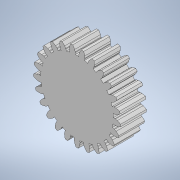
# Autodesk Inventor part: ｍ2歯数25ギア8t
Saved by Autodesk Inventor 2020.2 (Build 242310000, 310)
## iProperties
Created: 2020-02-29
Part Number: ｍ2歯数25ギア8t
Material: 一般
Document SubType Name: Modeling
Designer: aoyam
Density: 1 g/cm^3
Appearance: 既定
Author: aoyam
Autodesk Inventor part; units mm, degrees
ref_plane "YZ Plane" through (0, 0, 0) normal (1, 0, 0) x (0, 1, 0)
ref_plane "XZ Plane" through (0, 0, 0) normal (0, 1, 0) x (-1, 0, 0)
ref_plane "XY Plane" through (0, 0, 0) normal (0, 0, 1) x (1, 0, 0)
sketch "スケッチ1" plane through (0, 0, 0) normal (0, 0, 1) x (1, 0, 0)
  arc A0 (3.1095, 14.9151) -> (3.0807, 14.7407) centre (4.2203, 14.6422) ccw
  arc A1 (3.2924, 15.4594) -> (3.1095, 14.9151) centre (6.1695, 14.1895) ccw
  arc A2 (3.8523, 16.442) -> (3.2924, 15.4594) centre (8.2697, 13.2741) ccw
  arc A3 (1.9552, 14.7407) -> (1.9264, 14.9151) centre (0.8156, 14.6422) ccw
  arc A4 (1.9264, 14.9151) -> (1.7434, 15.4594) centre (-1.1336, 14.1895) ccw
  arc A5 (1.7434, 15.4594) -> (1.1836, 16.442) centre (-3.2338, 13.2741) ccw
  arc A6 (3.0569, 14.2452) -> (1.979, 14.2452) centre (2.5179, 3.0081) ccw
  arc A7 (1.1836, 16.442) -> (0.4695, 16.3518) centre (2.5179, 3.0081) ccw
  line L0 (3.0569, 14.2452) -> (3.0807, 14.7407)
  line L1 (1.979, 14.2452) -> (1.9552, 14.7407)
  arc A8 (3.1095, 14.9151) -> (3.0807, 14.7407) centre (4.2203, 14.6422) ccw
  arc A9 (3.2924, 15.4594) -> (3.1095, 14.9151) centre (6.1695, 14.1895) ccw
  arc A10 (3.8523, 16.442) -> (3.2924, 15.4594) centre (8.2697, 13.2741) ccw
  arc A11 (1.9552, 14.7407) -> (1.9264, 14.9151) centre (0.8156, 14.6422) ccw
  arc A12 (1.9264, 14.9151) -> (1.7434, 15.4594) centre (-1.1336, 14.1895) ccw
  arc A13 (1.7434, 15.4594) -> (1.1836, 16.442) centre (-3.2338, 13.2741) ccw
  arc A14 (3.0569, 14.2452) -> (1.979, 14.2452) centre (2.5179, 3.0081) ccw
  arc A15 (1.1836, 16.442) -> (0.4695, 16.3518) centre (2.5179, 3.0081) ccw
  line L2 (3.0569, 14.2452) -> (3.0807, 14.7407)
  line L3 (1.979, 14.2452) -> (1.9552, 14.7407)
  arc A16 (-0.9449, 14.2322) -> (-1.0161, 14.3939) centre (-2.0242, 13.8533) ccw
  arc A17 (-0.9449, 14.2322) -> (-1.0161, 14.3939) centre (-2.0242, 13.8533) ccw
  line L4 (-0.7987, 13.7581) -> (-0.9449, 14.2322)
  line L5 (-0.7987, 13.7581) -> (-0.9449, 14.2322)
  arc A18 (0.1297, 14.6881) -> (0.1452, 14.5121) centre (1.2735, 14.7) ccw
  arc A19 (0.1716, 15.2609) -> (0.1297, 14.6881) centre (3.2741, 14.7463) ccw
  arc A20 (0.4695, 16.3518) -> (0.1716, 15.2609) centre (5.5359, 14.3819) ccw
  line L6 (0.2454, 14.0262) -> (0.1452, 14.5121)
  line L7 (0.2454, 14.0262) -> (0.1452, 14.5121)
  arc A21 (0.1297, 14.6881) -> (0.1452, 14.5121) centre (1.2735, 14.7) ccw
  arc A22 (0.1716, 15.2609) -> (0.1297, 14.6881) centre (3.2741, 14.7463) ccw
  arc A23 (0.4695, 16.3518) -> (0.1716, 15.2609) centre (5.5359, 14.3819) ccw
  arc A24 (-1.0161, 14.3939) -> (-1.3287, 14.8756) centre (-3.7996, 12.9301) ccw
  arc A25 (-1.0161, 14.3939) -> (-1.3287, 14.8756) centre (-3.7996, 12.9301) ccw
  arc A26 (-1.3287, 14.8756) -> (-2.1154, 15.6881) centre (-5.6061, 11.5211) ccw
  arc A27 (-2.1154, 15.6881) -> (-2.7846, 15.4231) centre (2.5179, 3.0081) ccw
  arc A28 (-2.1154, 15.6881) -> (-2.7846, 15.4231) centre (2.5179, 3.0081) ccw
  arc A29 (-1.3287, 14.8756) -> (-2.1154, 15.6881) centre (-5.6061, 11.5211) ccw
  arc A30 (0.2454, 14.0262) -> (-0.7987, 13.7581) centre (2.5179, 3.0081) ccw
  arc A31 (0.2454, 14.0262) -> (-0.7987, 13.7581) centre (2.5179, 3.0081) ccw
  arc A32 (-3.6275, 13.0184) -> (-3.7367, 13.1573) centre (-4.5786, 12.383) ccw
  arc A33 (-3.6275, 13.0184) -> (-3.7367, 13.1573) centre (-4.5786, 12.383) ccw
  line L8 (-3.3679, 12.5956) -> (-3.6275, 13.0184)
  line L9 (-3.3679, 12.5956) -> (-3.6275, 13.0184)
  arc A34 (-2.6999, 13.7272) -> (-2.6412, 13.5606) centre (-1.5951, 14.0232) ccw
  arc A35 (-2.8019, 14.2924) -> (-2.6999, 13.7272) centre (0.3311, 14.5656) ccw
  arc A36 (-2.7846, 15.4231) -> (-2.8019, 14.2924) centre (2.6125, 14.7751) ccw
  line L10 (-2.4233, 13.1149) -> (-2.6412, 13.5606)
  line L11 (-2.4233, 13.1149) -> (-2.6412, 13.5606)
  arc A37 (-2.6999, 13.7272) -> (-2.6412, 13.5606) centre (-1.5951, 14.0232) ccw
  arc A38 (-2.8019, 14.2924) -> (-2.6999, 13.7272) centre (0.3311, 14.5656) ccw
  arc A39 (-2.7846, 15.4231) -> (-2.8019, 14.2924) centre (2.6125, 14.7751) ccw
  arc A40 (-3.7367, 13.1573) -> (-4.1592, 13.5462) centre (-6.0686, 11.0473) ccw
  arc A41 (-3.7367, 13.1573) -> (-4.1592, 13.5462) centre (-6.0686, 11.0473) ccw
  arc A42 (-4.1592, 13.5462) -> (-5.1232, 14.1374) centre (-7.468, 9.2333) ccw
  arc A43 (-5.1232, 14.1374) -> (-5.7055, 13.7144) centre (2.5179, 3.0081) ccw
  arc A44 (-5.1232, 14.1374) -> (-5.7055, 13.7144) centre (2.5179, 3.0081) ccw
  arc A45 (-4.1592, 13.5462) -> (-5.1232, 14.1374) centre (-7.468, 9.2333) ccw
  arc A46 (-2.4233, 13.1149) -> (-3.3679, 12.5956) centre (2.5179, 3.0081) ccw
  arc A47 (-2.4233, 13.1149) -> (-3.3679, 12.5956) centre (2.5179, 3.0081) ccw
  arc A48 (-5.9238, 11.1756) -> (-6.0642, 11.283) centre (-6.6871, 10.3236) ccw
  arc A49 (-5.9238, 11.1756) -> (-6.0642, 11.283) centre (-6.6871, 10.3236) ccw
  line L12 (-5.5673, 10.8306) -> (-5.9238, 11.1756)
  line L13 (-5.5673, 10.8306) -> (-5.9238, 11.1756)
  arc A50 (-5.2017, 12.0928) -> (-5.1034, 11.9461) centre (-4.2052, 12.6543) ccw
  arc A51 (-5.441, 12.6149) -> (-5.2017, 12.0928) centre (-2.4744, 13.6586) ccw
  arc A52 (-5.7055, 13.7144) -> (-5.441, 12.6149) centre (-0.3168, 14.429) ccw
  line L14 (-4.7815, 11.5685) -> (-5.1034, 11.9461)
  line L15 (-4.7815, 11.5685) -> (-5.1034, 11.9461)
  arc A53 (-5.2017, 12.0928) -> (-5.1034, 11.9461) centre (-4.2052, 12.6543) ccw
  arc A54 (-5.441, 12.6149) -> (-5.2017, 12.0928) centre (-2.4744, 13.6586) ccw
  arc A55 (-5.7055, 13.7144) -> (-5.441, 12.6149) centre (-0.3168, 14.429) ccw
  arc A56 (-6.0642, 11.283) -> (-6.5702, 11.5545) centre (-7.7981, 8.6593) ccw
  arc A57 (-6.0642, 11.283) -> (-6.5702, 11.5545) centre (-7.7981, 8.6593) ccw
  arc A58 (-6.5702, 11.5545) -> (-7.6509, 11.8875) centre (-8.7024, 6.5543) ccw
  arc A59 (-7.6509, 11.8875) -> (-8.1097, 11.333) centre (2.5179, 3.0081) ccw
  arc A60 (-7.6509, 11.8875) -> (-8.1097, 11.333) centre (2.5179, 3.0081) ccw
  arc A61 (-6.5702, 11.5545) -> (-7.6509, 11.8875) centre (-8.7024, 6.5543) ccw
  arc A62 (-4.7815, 11.5685) -> (-5.5673, 10.8306) centre (2.5179, 3.0081) ccw
  arc A63 (-4.7815, 11.5685) -> (-5.5673, 10.8306) centre (2.5179, 3.0081) ccw
  arc A64 (-7.6898, 8.8196) -> (-7.8524, 8.8887) centre (-8.2172, 7.8046) ccw
  arc A65 (-7.6898, 8.8196) -> (-7.8524, 8.8887) centre (-8.2172, 7.8046) ccw
  line L16 (-7.2586, 8.5741) -> (-7.6898, 8.8196)
  line L17 (-7.2586, 8.5741) -> (-7.6898, 8.8196)
  arc A66 (-7.2185, 9.8876) -> (-7.0867, 9.7699) centre (-6.3929, 10.6792) ccw
  arc A67 (-7.5801, 10.3338) -> (-7.2185, 9.8876) centre (-4.9662, 12.0825) ccw
  arc A68 (-8.1097, 11.333) -> (-7.5801, 10.3338) centre (-3.068, 13.3652) ccw
  line L18 (-6.681, 9.4843) -> (-7.0867, 9.7699)
  line L19 (-6.681, 9.4843) -> (-7.0867, 9.7699)
  arc A69 (-7.2185, 9.8876) -> (-7.0867, 9.7699) centre (-6.3929, 10.6792) ccw
  arc A70 (-7.5801, 10.3338) -> (-7.2185, 9.8876) centre (-4.9662, 12.0825) ccw
  arc A71 (-8.1097, 11.333) -> (-7.5801, 10.3338) centre (-3.068, 13.3652) ccw
  arc A72 (-7.8524, 8.8887) -> (-8.4101, 9.0259) centre (-8.8794, 5.9163) ccw
  arc A73 (-7.8524, 8.8887) -> (-8.4101, 9.0259) centre (-8.8794, 5.9163) ccw
  arc A74 (-8.4101, 9.0259) -> (-9.5397, 9.0797) centre (-9.2318, 3.6525) ccw
  arc A75 (-9.5397, 9.0797) -> (-9.8461, 8.4284) centre (2.5179, 3.0081) ccw
  arc A76 (-9.5397, 9.0797) -> (-9.8461, 8.4284) centre (2.5179, 3.0081) ccw
  arc A77 (-8.4101, 9.0259) -> (-9.5397, 9.0797) centre (-9.2318, 3.6525) ccw
  arc A78 (-6.681, 9.4843) -> (-7.2586, 8.5741) centre (2.5179, 3.0081) ccw
  arc A79 (-6.681, 9.4843) -> (-7.2586, 8.5741) centre (2.5179, 3.0081) ccw
  arc A80 (-8.8144, 6.0985) -> (-8.9891, 6.125) centre (-9.0728, 4.9842) ccw
  arc A81 (-8.8144, 6.0985) -> (-8.9891, 6.125) centre (-9.0728, 4.9842) ccw
  line L20 (-8.3357, 5.9679) -> (-8.8144, 6.0985)
  line L21 (-8.3357, 5.9679) -> (-8.8144, 6.0985)
  arc A82 (-8.6235, 7.2501) -> (-8.4666, 7.1689) centre (-8.0207, 8.2222) ccw
  arc A83 (-9.0847, 7.5923) -> (-8.6235, 7.2501) centre (-6.9878, 9.9362) ccw
  arc A84 (-9.8461, 8.4284) -> (-9.0847, 7.5923) centre (-5.4682, 11.6507) ccw
  line L22 (-8.0026, 6.9931) -> (-8.4666, 7.1689)
  line L23 (-8.0026, 6.9931) -> (-8.4666, 7.1689)
  arc A85 (-8.6235, 7.2501) -> (-8.4666, 7.1689) centre (-8.0207, 8.2222) ccw
  arc A86 (-9.0847, 7.5923) -> (-8.6235, 7.2501) centre (-6.9878, 9.9362) ccw
  arc A87 (-9.8461, 8.4284) -> (-9.0847, 7.5923) centre (-5.4682, 11.6507) ccw
  arc A88 (-8.9891, 6.125) -> (-9.5633, 6.1192) centre (-9.2446, 2.9905) ccw
  arc A89 (-8.9891, 6.125) -> (-9.5633, 6.1192) centre (-9.2446, 2.9905) ccw
  arc A90 (-9.5633, 6.1192) -> (-10.6708, 5.8903) centre (-9.023, 0.7102) ccw
  arc A91 (-10.6708, 5.8903) -> (-10.8057, 5.1833) centre (2.5179, 3.0081) ccw
  arc A92 (-10.6708, 5.8903) -> (-10.8057, 5.1833) centre (2.5179, 3.0081) ccw
  arc A93 (-9.5633, 6.1192) -> (-10.6708, 5.8903) centre (-9.023, 0.7102) ccw
  arc A94 (-8.0026, 6.9931) -> (-8.3357, 5.9679) centre (2.5179, 3.0081) ccw
  arc A95 (-8.0026, 6.9931) -> (-8.3357, 5.9679) centre (2.5179, 3.0081) ccw
  arc A96 (-9.2269, 3.1831) -> (-9.4027, 3.1654) centre (-9.2001, 2.0396) ccw
  arc A97 (-9.2269, 3.1831) -> (-9.4027, 3.1654) centre (-9.2001, 2.0396) ccw
  line L24 (-8.7308, 3.1757) -> (-9.2269, 3.1831)
  line L25 (-8.7308, 3.1757) -> (-9.2269, 3.1831)
  arc A98 (-9.3284, 4.3461) -> (-9.1562, 4.3064) centre (-8.9863, 5.4375) ccw
  arc A99 (-9.8602, 4.5629) -> (-9.3284, 4.3461) centre (-8.4121, 7.3545) ccw
  arc A100 (-10.8057, 5.1833) -> (-9.8602, 4.5629) centre (-7.3666, 9.3931) ccw
  line L26 (-8.6631, 4.2516) -> (-9.1562, 4.3064)
  line L27 (-8.6631, 4.2516) -> (-9.1562, 4.3064)
  arc A101 (-9.3284, 4.3461) -> (-9.1562, 4.3064) centre (-8.9863, 5.4375) ccw
  arc A102 (-9.8602, 4.5629) -> (-9.3284, 4.3461) centre (-8.4121, 7.3545) ccw
  arc A103 (-10.8057, 5.1833) -> (-9.8602, 4.5629) centre (-7.3666, 9.3931) ccw
  arc A104 (-9.4027, 3.1654) -> (-9.9575, 3.0169) centre (-8.8707, 0.0658) ccw
  arc A105 (-9.4027, 3.1654) -> (-9.9575, 3.0169) centre (-8.8707, 0.0658) ccw
  arc A106 (-9.9575, 3.0169) -> (-10.9732, 2.5199) centre (-8.0889, -2.0877) ccw
  arc A107 (-10.9732, 2.5199) -> (-10.928, 1.8015) centre (2.5179, 3.0081) ccw
  arc A108 (-10.9732, 2.5199) -> (-10.928, 1.8015) centre (2.5179, 3.0081) ccw
  arc A109 (-9.9575, 3.0169) -> (-10.9732, 2.5199) centre (-8.0889, -2.0877) ccw
  arc A110 (-8.6631, 4.2516) -> (-8.7308, 3.1757) centre (2.5179, 3.0081) ccw
  arc A111 (-8.6631, 4.2516) -> (-8.7308, 3.1757) centre (2.5179, 3.0081) ccw
  arc A112 (-8.9015, 0.2568) -> (-9.0673, 0.1959) centre (-8.5911, -0.8441) ccw
  arc A113 (-8.9015, 0.2568) -> (-9.0673, 0.1959) centre (-8.5911, -0.8441) ccw
  line L28 (-8.4191, 0.373) -> (-8.9015, 0.2568)
  line L29 (-8.4191, 0.373) -> (-8.9015, 0.2568)
  arc A114 (-9.289, 1.358) -> (-9.1124, 1.3624) centre (-9.229, 2.5002) ccw
  arc A115 (-9.858, 1.4357) -> (-9.289, 1.358) centre (-9.1497, 4.4998) ccw
  arc A116 (-10.928, 1.8015) -> (-9.858, 1.4357) centre (-8.644, 6.7343) ccw
  line L30 (-8.6211, 1.4319) -> (-9.1124, 1.3624)
  line L31 (-8.6211, 1.4319) -> (-9.1124, 1.3624)
  arc A117 (-9.289, 1.358) -> (-9.1124, 1.3624) centre (-9.229, 2.5002) ccw
  arc A118 (-9.858, 1.4357) -> (-9.289, 1.358) centre (-9.1497, 4.4998) ccw
  arc A119 (-10.928, 1.8015) -> (-9.858, 1.4357) centre (-8.644, 6.7343) ccw
  arc A120 (-9.0673, 0.1959) -> (-9.5677, -0.0859) centre (-7.7812, -2.674) ccw
  arc A121 (-9.0673, 0.1959) -> (-9.5677, -0.0859) centre (-7.7812, -2.674) ccw
  arc A122 (-9.5677, -0.0859) -> (-10.428, -0.8199) centre (-6.4884, -4.5654) ccw
  arc A123 (-10.428, -0.8199) -> (-10.2056, -1.5044) centre (2.5179, 3.0081) ccw
  arc A124 (-10.428, -0.8199) -> (-10.2056, -1.5044) centre (2.5179, 3.0081) ccw
  arc A125 (-9.5677, -0.0859) -> (-10.428, -0.8199) centre (-6.4884, -4.5654) ccw
  arc A126 (-8.6211, 1.4319) -> (-8.4191, 0.373) centre (2.5179, 3.0081) ccw
  arc A127 (-8.6211, 1.4319) -> (-8.4191, 0.373) centre (2.5179, 3.0081) ccw
  arc A128 (-7.8585, -2.4966) -> (-8.004, -2.5969) centre (-7.2841, -3.4858) ccw
  arc A129 (-7.8585, -2.4966) -> (-8.004, -2.5969) centre (-7.2841, -3.4858) ccw
  line L32 (-7.4202, -2.2641) -> (-7.8585, -2.4966)
  line L33 (-7.4202, -2.2641) -> (-7.8585, -2.4966)
  arc A130 (-8.5077, -1.5264) -> (-8.3377, -1.4783) centre (-8.7337, -0.4052) ccw
  arc A131 (-9.0782, -1.5927) -> (-8.5077, -1.5264) centre (-9.1541, 1.5513) ccw
  arc A132 (-10.2056, -1.5044) -> (-9.0782, -1.5927) centre (-9.22, 3.8413) ccw
  line L34 (-7.8792, -1.2888) -> (-8.3377, -1.4783)
  line L35 (-7.8792, -1.2888) -> (-8.3377, -1.4783)
  arc A133 (-8.5077, -1.5264) -> (-8.3377, -1.4783) centre (-8.7337, -0.4052) ccw
  arc A134 (-9.0782, -1.5927) -> (-8.5077, -1.5264) centre (-9.1541, 1.5513) ccw
  arc A135 (-10.2056, -1.5044) -> (-9.0782, -1.5927) centre (-9.22, 3.8413) ccw
  arc A136 (-8.004, -2.5969) -> (-8.4186, -2.9942) centre (-6.0446, -5.0568) ccw
  arc A137 (-8.004, -2.5969) -> (-8.4186, -2.9942) centre (-6.0446, -5.0568) ccw
  arc A138 (-8.4186, -2.9942) -> (-9.0693, -3.9192) centre (-4.322, -6.5673) ccw
  arc A139 (-9.0693, -3.9192) -> (-8.6836, -4.5269) centre (2.5179, 3.0081) ccw
  arc A140 (-9.0693, -3.9192) -> (-8.6836, -4.5269) centre (2.5179, 3.0081) ccw
  arc A141 (-8.4186, -2.9942) -> (-9.0693, -3.9192) centre (-4.322, -6.5673) ccw
  arc A142 (-7.8792, -1.2888) -> (-7.4202, -2.2641) centre (2.5179, 3.0081) ccw
  arc A143 (-7.8792, -1.2888) -> (-7.4202, -2.2641) centre (2.5179, 3.0081) ccw
  arc A144 (-6.1635, -4.9042) -> (-6.2795, -5.0375) centre (-5.3612, -5.7194) ccw
  arc A145 (-6.1635, -4.9042) -> (-6.2795, -5.0375) centre (-5.3612, -5.7194) ccw
  line L36 (-5.7968, -4.57) -> (-6.1635, -4.9042)
  line L37 (-5.7968, -4.57) -> (-6.1635, -4.9042)
  arc A146 (-7.0336, -4.1259) -> (-6.8809, -4.037) centre (-7.5314, -3.0961) ccw
  arc A147 (-7.5697, -4.332) -> (-7.0336, -4.1259) centre (-8.4251, -1.3057) ccw
  arc A148 (-8.6836, -4.5269) -> (-7.5697, -4.332) centre (-9.0584, 0.8961) ccw
  line L38 (-6.4839, -3.7394) -> (-6.8809, -4.037)
  line L39 (-6.4839, -3.7394) -> (-6.8809, -4.037)
  arc A149 (-7.0336, -4.1259) -> (-6.8809, -4.037) centre (-7.5314, -3.0961) ccw
  arc A150 (-7.5697, -4.332) -> (-7.0336, -4.1259) centre (-8.4251, -1.3057) ccw
  arc A151 (-8.6836, -4.5269) -> (-7.5697, -4.332) centre (-9.0584, 0.8961) ccw
  arc A152 (-6.2795, -5.0375) -> (-6.5823, -5.5255) centre (-3.7699, -6.9328) ccw
  arc A153 (-6.2795, -5.0375) -> (-6.5823, -5.5255) centre (-3.7699, -6.9328) ccw
  arc A154 (-6.5823, -5.5255) -> (-6.9825, -6.5832) centre (-1.7258, -7.9675) ccw
  arc A155 (-6.9825, -6.5832) -> (-6.4578, -7.0759) centre (2.5179, 3.0081) ccw
  arc A156 (-6.9825, -6.5832) -> (-6.4578, -7.0759) centre (2.5179, 3.0081) ccw
  arc A157 (-6.5823, -5.5255) -> (-6.9825, -6.5832) centre (-1.7258, -7.9675) ccw
  arc A158 (-6.4839, -3.7394) -> (-5.7968, -4.57) centre (2.5179, 3.0081) ccw
  arc A159 (-6.4839, -3.7394) -> (-5.7968, -4.57) centre (2.5179, 3.0081) ccw
  arc A160 (-3.9231, -6.8146) -> (-4.0023, -6.9726) centre (-2.9432, -7.4047) ccw
  arc A161 (-3.9231, -6.8146) -> (-4.0023, -6.9726) centre (-2.9432, -7.4047) ccw
  line L40 (-3.651, -6.3997) -> (-3.9231, -6.8146)
  line L41 (-3.651, -6.3997) -> (-3.9231, -6.8146)
  arc A162 (-4.9594, -6.2772) -> (-4.8336, -6.1531) centre (-5.6976, -5.4035) ccw
  arc A163 (-5.4274, -6.6101) -> (-4.9594, -6.2772) centre (-7.0085, -3.8916) ccw
  arc A164 (-6.4578, -7.0759) -> (-5.4274, -6.6101) centre (-8.1695, -1.9165) ccw
  line L42 (-4.5231, -5.7661) -> (-4.8336, -6.1531)
  line L43 (-4.5231, -5.7661) -> (-4.8336, -6.1531)
  arc A165 (-4.9594, -6.2772) -> (-4.8336, -6.1531) centre (-5.6976, -5.4035) ccw
  arc A166 (-5.4274, -6.6101) -> (-4.9594, -6.2772) centre (-7.0085, -3.8916) ccw
  arc A167 (-6.4578, -7.0759) -> (-5.4274, -6.6101) centre (-8.1695, -1.9165) ccw
  arc A168 (-4.0023, -6.9726) -> (-4.1742, -7.5205) centre (-1.1002, -8.1842) ccw
  arc A169 (-4.0023, -6.9726) -> (-4.1742, -7.5205) centre (-1.1002, -8.1842) ccw
  arc A170 (-4.1742, -7.5205) -> (-4.2988, -8.6445) centre (1.137, -8.6781) ccw
  arc A171 (-4.2988, -8.6445) -> (-3.6681, -8.9912) centre (2.5179, 3.0081) ccw
  arc A172 (-4.2988, -8.6445) -> (-3.6681, -8.9912) centre (2.5179, 3.0081) ccw
  arc A173 (-4.1742, -7.5205) -> (-4.2988, -8.6445) centre (1.137, -8.6781) ccw
  arc A174 (-4.5231, -5.7661) -> (-3.651, -6.3997) centre (2.5179, 3.0081) ccw
  arc A175 (-4.5231, -5.7661) -> (-3.651, -6.3997) centre (2.5179, 3.0081) ccw
  arc A176 (-1.2779, -8.1078) -> (-1.3153, -8.2805) centre (-0.1821, -8.4357) ccw
  arc A177 (-1.2779, -8.1078) -> (-1.3153, -8.2805) centre (-0.1821, -8.4357) ccw
  line L44 (-1.1176, -7.6383) -> (-1.2779, -8.1078)
  line L45 (-1.1176, -7.6383) -> (-1.2779, -8.1078)
  arc A178 (-2.4153, -7.845) -> (-2.3244, -7.6935) centre (-3.3476, -7.1824) ccw
  arc A179 (-2.7858, -8.2838) -> (-2.4153, -7.845) centre (-4.9933, -6.0439) ccw
  arc A180 (-3.6681, -8.9912) -> (-2.7858, -8.2838) centre (-6.609, -4.4196) ccw
  line L46 (-2.1198, -7.2415) -> (-2.3244, -7.6935)
  line L47 (-2.1198, -7.2415) -> (-2.3244, -7.6935)
  arc A181 (-2.4153, -7.845) -> (-2.3244, -7.6935) centre (-3.3476, -7.1824) ccw
  arc A182 (-2.7858, -8.2838) -> (-2.4153, -7.845) centre (-4.9933, -6.0439) ccw
  arc A183 (-3.6681, -8.9912) -> (-2.7858, -8.2838) centre (-6.609, -4.4196) ccw
  arc A184 (-1.3153, -8.2805) -> (-1.3456, -8.854) centre (1.7969, -8.7324) ccw
  arc A185 (-1.3153, -8.2805) -> (-1.3456, -8.854) centre (1.7969, -8.7324) ccw
  arc A186 (-1.3456, -8.854) -> (-1.1867, -9.9737) centre (4.0866, -8.6543) ccw
  arc A187 (-1.1867, -9.9737) -> (-0.4896, -10.1526) centre (2.5179, 3.0081) ccw
  arc A188 (-1.1867, -9.9737) -> (-0.4896, -10.1526) centre (2.5179, 3.0081) ccw
  arc A189 (-1.3456, -8.854) -> (-1.1867, -9.9737) centre (4.0866, -8.6543) ccw
  arc A190 (-2.1198, -7.2415) -> (-1.1176, -7.6383) centre (2.5179, 3.0081) ccw
  arc A191 (-2.1198, -7.2415) -> (-1.1176, -7.6383) centre (2.5179, 3.0081) ccw
  arc A192 (1.6058, -8.7026) -> (1.6125, -8.8792) centre (2.7487, -8.7476) ccw
  arc A193 (1.6058, -8.7026) -> (1.6125, -8.8792) centre (2.7487, -8.7476) ccw
  line L48 (1.6443, -8.208) -> (1.6058, -8.7026)
  line L49 (1.6443, -8.208) -> (1.6058, -8.7026)
  arc A194 (0.4387, -8.7309) -> (0.4891, -8.5615) centre (-0.6291, -8.3209) ccw
  arc A195 (0.189, -9.248) -> (0.4387, -8.7309) centre (-2.5062, -7.6275) ccw
  arc A196 (-0.4896, -10.1526) -> (0.189, -9.248) centre (-4.4751, -6.4561) ccw
  line L50 (0.5748, -8.0728) -> (0.4891, -8.5615)
  line L51 (0.5748, -8.0728) -> (0.4891, -8.5615)
  arc A197 (0.4387, -8.7309) -> (0.4891, -8.5615) centre (-0.6291, -8.3209) ccw
  arc A198 (0.189, -9.248) -> (0.4387, -8.7309) centre (-2.5062, -7.6275) ccw
  arc A199 (-0.4896, -10.1526) -> (0.189, -9.248) centre (-4.4751, -6.4561) ccw
  arc A200 (1.6125, -8.8792) -> (1.7258, -9.4422) centre (4.7393, -8.5428) ccw
  arc A201 (1.6125, -8.8792) -> (1.7258, -9.4422) centre (4.7393, -8.5428) ccw
  arc A202 (1.7258, -9.4422) -> (2.1581, -10.4871) centre (6.9376, -7.8978) ccw
  arc A203 (2.1581, -10.4871) -> (2.8778, -10.4871) centre (2.5179, 3.0081) ccw
  arc A204 (2.1581, -10.4871) -> (2.8778, -10.4871) centre (2.5179, 3.0081) ccw
  arc A205 (1.7258, -9.4422) -> (2.1581, -10.4871) centre (6.9376, -7.8978) ccw
  arc A206 (0.5748, -8.0728) -> (1.6443, -8.208) centre (2.5179, 3.0081) ccw
  arc A207 (0.5748, -8.0728) -> (1.6443, -8.208) centre (2.5179, 3.0081) ccw
  arc A208 (4.5467, -8.5615) -> (4.5971, -8.7309) centre (5.665, -8.3209) ccw
  arc A209 (4.5467, -8.5615) -> (4.5971, -8.7309) centre (5.665, -8.3209) ccw
  line L52 (4.4611, -8.0728) -> (4.5467, -8.5615)
  line L53 (4.4611, -8.0728) -> (4.5467, -8.5615)
  arc A210 (3.4234, -8.8792) -> (3.4301, -8.7026) centre (2.2872, -8.7476) ccw
  arc A211 (3.3101, -9.4422) -> (3.4234, -8.8792) centre (0.2966, -8.5428) ccw
  arc A212 (2.8778, -10.4871) -> (3.3101, -9.4422) centre (-1.9018, -7.8978) ccw
  line L54 (3.3916, -8.208) -> (3.4301, -8.7026)
  line L55 (3.3916, -8.208) -> (3.4301, -8.7026)
  arc A213 (3.4234, -8.8792) -> (3.4301, -8.7026) centre (2.2872, -8.7476) ccw
  arc A214 (3.3101, -9.4422) -> (3.4234, -8.8792) centre (0.2966, -8.5428) ccw
  arc A215 (2.8778, -10.4871) -> (3.3101, -9.4422) centre (-1.9018, -7.8978) ccw
  arc A216 (4.5971, -8.7309) -> (4.8469, -9.248) centre (7.5421, -7.6275) ccw
  arc A217 (4.5971, -8.7309) -> (4.8469, -9.248) centre (7.5421, -7.6275) ccw
  arc A218 (4.8469, -9.248) -> (5.5255, -10.1526) centre (9.511, -6.4561) ccw
  arc A219 (5.5255, -10.1526) -> (6.2226, -9.9737) centre (2.5179, 3.0081) ccw
  arc A220 (5.5255, -10.1526) -> (6.2226, -9.9737) centre (2.5179, 3.0081) ccw
  arc A221 (4.8469, -9.248) -> (5.5255, -10.1526) centre (9.511, -6.4561) ccw
  arc A222 (3.3916, -8.208) -> (4.4611, -8.0728) centre (2.5179, 3.0081) ccw
  arc A223 (3.3916, -8.208) -> (4.4611, -8.0728) centre (2.5179, 3.0081) ccw
  arc A224 (7.3603, -7.6935) -> (7.4512, -7.845) centre (8.3835, -7.1824) ccw
  arc A225 (7.3603, -7.6935) -> (7.4512, -7.845) centre (8.3835, -7.1824) ccw
  line L56 (7.1557, -7.2415) -> (7.3603, -7.6935)
  line L57 (7.1557, -7.2415) -> (7.3603, -7.6935)
  arc A226 (6.3512, -8.2805) -> (6.3138, -8.1078) centre (5.218, -8.4357) ccw
  arc A227 (6.3815, -8.854) -> (6.3512, -8.2805) centre (3.239, -8.7324) ccw
  arc A228 (6.2226, -9.9737) -> (6.3815, -8.854) centre (0.9493, -8.6543) ccw
  line L58 (6.1535, -7.6383) -> (6.3138, -8.1078)
  line L59 (6.1535, -7.6383) -> (6.3138, -8.1078)
  arc A229 (6.3512, -8.2805) -> (6.3138, -8.1078) centre (5.218, -8.4357) ccw
  arc A230 (6.3815, -8.854) -> (6.3512, -8.2805) centre (3.239, -8.7324) ccw
  arc A231 (6.2226, -9.9737) -> (6.3815, -8.854) centre (0.9493, -8.6543) ccw
  arc A232 (7.4512, -7.845) -> (7.8217, -8.2838) centre (10.0292, -6.0439) ccw
  arc A233 (7.4512, -7.845) -> (7.8217, -8.2838) centre (10.0292, -6.0439) ccw
  arc A234 (7.8217, -8.2838) -> (8.704, -8.9912) centre (11.6449, -4.4196) ccw
  arc A235 (8.704, -8.9912) -> (9.3347, -8.6445) centre (2.5179, 3.0081) ccw
  arc A236 (8.704, -8.9912) -> (9.3347, -8.6445) centre (2.5179, 3.0081) ccw
  arc A237 (7.8217, -8.2838) -> (8.704, -8.9912) centre (11.6449, -4.4196) ccw
  arc A238 (6.1535, -7.6383) -> (7.1557, -7.2415) centre (2.5179, 3.0081) ccw
  arc A239 (6.1535, -7.6383) -> (7.1557, -7.2415) centre (2.5179, 3.0081) ccw
  arc A240 (9.8695, -6.1531) -> (9.9953, -6.2772) centre (10.7335, -5.4035) ccw
  arc A241 (9.8695, -6.1531) -> (9.9953, -6.2772) centre (10.7335, -5.4035) ccw
  line L60 (9.559, -5.7661) -> (9.8695, -6.1531)
  line L61 (9.559, -5.7661) -> (9.8695, -6.1531)
  arc A242 (9.0381, -6.9726) -> (8.959, -6.8146) centre (7.9791, -7.4047) ccw
  arc A243 (9.2101, -7.5205) -> (9.0381, -6.9726) centre (6.136, -8.1842) ccw
  arc A244 (9.3347, -8.6445) -> (9.2101, -7.5205) centre (3.8989, -8.6781) ccw
  line L62 (8.6869, -6.3997) -> (8.959, -6.8146)
  line L63 (8.6869, -6.3997) -> (8.959, -6.8146)
  arc A245 (9.0381, -6.9726) -> (8.959, -6.8146) centre (7.9791, -7.4047) ccw
  arc A246 (9.2101, -7.5205) -> (9.0381, -6.9726) centre (6.136, -8.1842) ccw
  arc A247 (9.3347, -8.6445) -> (9.2101, -7.5205) centre (3.8989, -8.6781) ccw
  arc A248 (9.9953, -6.2772) -> (10.4633, -6.6101) centre (12.0444, -3.8916) ccw
  arc A249 (9.9953, -6.2772) -> (10.4633, -6.6101) centre (12.0444, -3.8916) ccw
  arc A250 (10.4633, -6.6101) -> (11.4937, -7.0759) centre (13.2054, -1.9165) ccw
  arc A251 (11.4937, -7.0759) -> (12.0184, -6.5832) centre (2.5179, 3.0081) ccw
  arc A252 (11.4937, -7.0759) -> (12.0184, -6.5832) centre (2.5179, 3.0081) ccw
  arc A253 (10.4633, -6.6101) -> (11.4937, -7.0759) centre (13.2054, -1.9165) ccw
  arc A254 (8.6869, -6.3997) -> (9.559, -5.7661) centre (2.5179, 3.0081) ccw
  arc A255 (8.6869, -6.3997) -> (9.559, -5.7661) centre (2.5179, 3.0081) ccw
  arc A256 (11.9168, -4.037) -> (12.0695, -4.1259) centre (12.5672, -3.0961) ccw
  arc A257 (11.9168, -4.037) -> (12.0695, -4.1259) centre (12.5672, -3.0961) ccw
  line L64 (11.5198, -3.7394) -> (11.9168, -4.037)
  line L65 (11.5198, -3.7394) -> (11.9168, -4.037)
  arc A258 (11.3154, -5.0375) -> (11.1994, -4.9042) centre (10.3971, -5.7194) ccw
  arc A259 (11.6182, -5.5255) -> (11.3154, -5.0375) centre (8.8058, -6.9328) ccw
  arc A260 (12.0184, -6.5832) -> (11.6182, -5.5255) centre (6.7617, -7.9675) ccw
  line L66 (10.8327, -4.57) -> (11.1994, -4.9042)
  line L67 (10.8327, -4.57) -> (11.1994, -4.9042)
  arc A261 (11.3154, -5.0375) -> (11.1994, -4.9042) centre (10.3971, -5.7194) ccw
  arc A262 (11.6182, -5.5255) -> (11.3154, -5.0375) centre (8.8058, -6.9328) ccw
  arc A263 (12.0184, -6.5832) -> (11.6182, -5.5255) centre (6.7617, -7.9675) ccw
  arc A264 (12.0695, -4.1259) -> (12.6056, -4.332) centre (13.461, -1.3057) ccw
  arc A265 (12.0695, -4.1259) -> (12.6056, -4.332) centre (13.461, -1.3057) ccw
  arc A266 (12.6056, -4.332) -> (13.7195, -4.5269) centre (14.0943, 0.8961) ccw
  arc A267 (13.7195, -4.5269) -> (14.1051, -3.9192) centre (2.5179, 3.0081) ccw
  arc A268 (13.7195, -4.5269) -> (14.1051, -3.9192) centre (2.5179, 3.0081) ccw
  arc A269 (12.6056, -4.332) -> (13.7195, -4.5269) centre (14.0943, 0.8961) ccw
  arc A270 (10.8327, -4.57) -> (11.5198, -3.7394) centre (2.5179, 3.0081) ccw
  arc A271 (10.8327, -4.57) -> (11.5198, -3.7394) centre (2.5179, 3.0081) ccw
  arc A272 (13.3736, -1.4783) -> (13.5436, -1.5264) centre (13.7696, -0.4052) ccw
  arc A273 (13.3736, -1.4783) -> (13.5436, -1.5264) centre (13.7696, -0.4052) ccw
  line L68 (12.915, -1.2888) -> (13.3736, -1.4783)
  line L69 (12.915, -1.2888) -> (13.3736, -1.4783)
  arc A274 (13.0399, -2.5969) -> (12.8944, -2.4966) centre (12.32, -3.4858) ccw
  arc A275 (13.4545, -2.9942) -> (13.0399, -2.5969) centre (11.0804, -5.0568) ccw
  arc A276 (14.1051, -3.9192) -> (13.4545, -2.9942) centre (9.3579, -6.5673) ccw
  line L70 (12.4561, -2.2641) -> (12.8944, -2.4966)
  line L71 (12.4561, -2.2641) -> (12.8944, -2.4966)
  arc A277 (13.0399, -2.5969) -> (12.8944, -2.4966) centre (12.32, -3.4858) ccw
  arc A278 (13.4545, -2.9942) -> (13.0399, -2.5969) centre (11.0804, -5.0568) ccw
  arc A279 (14.1051, -3.9192) -> (13.4545, -2.9942) centre (9.3579, -6.5673) ccw
  arc A280 (13.5436, -1.5264) -> (14.114, -1.5927) centre (14.1899, 1.5513) ccw
  arc A281 (13.5436, -1.5264) -> (14.114, -1.5927) centre (14.1899, 1.5513) ccw
  arc A282 (14.114, -1.5927) -> (15.2414, -1.5044) centre (14.2558, 3.8413) ccw
  arc A283 (15.2414, -1.5044) -> (15.4638, -0.8199) centre (2.5179, 3.0081) ccw
  arc A284 (15.2414, -1.5044) -> (15.4638, -0.8199) centre (2.5179, 3.0081) ccw
  arc A285 (14.114, -1.5927) -> (15.2414, -1.5044) centre (14.2558, 3.8413) ccw
  arc A286 (12.4561, -2.2641) -> (12.915, -1.2888) centre (2.5179, 3.0081) ccw
  arc A287 (12.4561, -2.2641) -> (12.915, -1.2888) centre (2.5179, 3.0081) ccw
  arc A288 (14.1482, 1.3624) -> (14.3249, 1.358) centre (14.2649, 2.5002) ccw
  arc A289 (14.1482, 1.3624) -> (14.3249, 1.358) centre (14.2649, 2.5002) ccw
  line L72 (13.657, 1.4319) -> (14.1482, 1.3624)
  line L73 (13.657, 1.4319) -> (14.1482, 1.3624)
  arc A290 (14.1032, 0.1959) -> (13.9373, 0.2568) centre (13.627, -0.8441) ccw
  arc A291 (14.6036, -0.0859) -> (14.1032, 0.1959) centre (12.8171, -2.674) ccw
  arc A292 (15.4638, -0.8199) -> (14.6036, -0.0859) centre (11.5243, -4.5654) ccw
  line L74 (13.455, 0.373) -> (13.9373, 0.2568)
  line L75 (13.455, 0.373) -> (13.9373, 0.2568)
  arc A293 (14.1032, 0.1959) -> (13.9373, 0.2568) centre (13.627, -0.8441) ccw
  arc A294 (14.6036, -0.0859) -> (14.1032, 0.1959) centre (12.8171, -2.674) ccw
  arc A295 (15.4638, -0.8199) -> (14.6036, -0.0859) centre (11.5243, -4.5654) ccw
  arc A296 (14.3249, 1.358) -> (14.8939, 1.4357) centre (14.1855, 4.4998) ccw
  arc A297 (14.3249, 1.358) -> (14.8939, 1.4357) centre (14.1855, 4.4998) ccw
  arc A298 (14.8939, 1.4357) -> (15.9639, 1.8015) centre (13.6799, 6.7343) ccw
  arc A299 (15.9639, 1.8015) -> (16.0091, 2.5199) centre (2.5179, 3.0081) ccw
  arc A300 (15.9639, 1.8015) -> (16.0091, 2.5199) centre (2.5179, 3.0081) ccw
  arc A301 (14.8939, 1.4357) -> (15.9639, 1.8015) centre (13.6799, 6.7343) ccw
  arc A302 (13.455, 0.373) -> (13.657, 1.4319) centre (2.5179, 3.0081) ccw
  arc A303 (13.455, 0.373) -> (13.657, 1.4319) centre (2.5179, 3.0081) ccw
  arc A304 (14.1921, 4.3064) -> (14.3643, 4.3461) centre (14.0222, 5.4375) ccw
  arc A305 (14.1921, 4.3064) -> (14.3643, 4.3461) centre (14.0222, 5.4375) ccw
  line L76 (13.699, 4.2516) -> (14.1921, 4.3064)
  line L77 (13.699, 4.2516) -> (14.1921, 4.3064)
  arc A306 (14.4386, 3.1654) -> (14.2628, 3.1831) centre (14.236, 2.0396) ccw
  arc A307 (14.9934, 3.0169) -> (14.4386, 3.1654) centre (13.9066, 0.0658) ccw
  arc A308 (16.0091, 2.5199) -> (14.9934, 3.0169) centre (13.1248, -2.0877) ccw
  line L78 (13.7667, 3.1757) -> (14.2628, 3.1831)
  line L79 (13.7667, 3.1757) -> (14.2628, 3.1831)
  arc A309 (14.4386, 3.1654) -> (14.2628, 3.1831) centre (14.236, 2.0396) ccw
  arc A310 (14.9934, 3.0169) -> (14.4386, 3.1654) centre (13.9066, 0.0658) ccw
  arc A311 (16.0091, 2.5199) -> (14.9934, 3.0169) centre (13.1248, -2.0877) ccw
  arc A312 (14.3643, 4.3461) -> (14.8961, 4.5629) centre (13.448, 7.3545) ccw
  arc A313 (14.3643, 4.3461) -> (14.8961, 4.5629) centre (13.448, 7.3545) ccw
  arc A314 (14.8961, 4.5629) -> (15.8415, 5.1833) centre (12.4025, 9.3931) ccw
  arc A315 (15.8415, 5.1833) -> (15.7067, 5.8903) centre (2.5179, 3.0081) ccw
  arc A316 (15.8415, 5.1833) -> (15.7067, 5.8903) centre (2.5179, 3.0081) ccw
  arc A317 (14.8961, 4.5629) -> (15.8415, 5.1833) centre (12.4025, 9.3931) ccw
  arc A318 (13.7667, 3.1757) -> (13.699, 4.2516) centre (2.5179, 3.0081) ccw
  arc A319 (13.7667, 3.1757) -> (13.699, 4.2516) centre (2.5179, 3.0081) ccw
  arc A320 (13.5025, 7.1689) -> (13.6594, 7.2501) centre (13.0566, 8.2222) ccw
  arc A321 (13.5025, 7.1689) -> (13.6594, 7.2501) centre (13.0566, 8.2222) ccw
  line L80 (13.0385, 6.9931) -> (13.5025, 7.1689)
  line L81 (13.0385, 6.9931) -> (13.5025, 7.1689)
  arc A322 (14.025, 6.125) -> (13.8503, 6.0985) centre (14.1087, 4.9842) ccw
  arc A323 (14.5992, 6.1192) -> (14.025, 6.125) centre (14.2805, 2.9905) ccw
  arc A324 (15.7067, 5.8903) -> (14.5992, 6.1192) centre (14.0589, 0.7102) ccw
  line L82 (13.3716, 5.9679) -> (13.8503, 6.0985)
  line L83 (13.3716, 5.9679) -> (13.8503, 6.0985)
  arc A325 (14.025, 6.125) -> (13.8503, 6.0985) centre (14.1087, 4.9842) ccw
  arc A326 (14.5992, 6.1192) -> (14.025, 6.125) centre (14.2805, 2.9905) ccw
  arc A327 (15.7067, 5.8903) -> (14.5992, 6.1192) centre (14.0589, 0.7102) ccw
  arc A328 (13.6594, 7.2501) -> (14.1206, 7.5923) centre (12.0237, 9.9362) ccw
  arc A329 (13.6594, 7.2501) -> (14.1206, 7.5923) centre (12.0237, 9.9362) ccw
  arc A330 (14.1206, 7.5923) -> (14.882, 8.4284) centre (10.5041, 11.6507) ccw
  arc A331 (14.882, 8.4284) -> (14.5755, 9.0797) centre (2.5179, 3.0081) ccw
  arc A332 (14.882, 8.4284) -> (14.5755, 9.0797) centre (2.5179, 3.0081) ccw
  arc A333 (14.1206, 7.5923) -> (14.882, 8.4284) centre (10.5041, 11.6507) ccw
  arc A334 (13.3716, 5.9679) -> (13.0385, 6.9931) centre (2.5179, 3.0081) ccw
  arc A335 (13.3716, 5.9679) -> (13.0385, 6.9931) centre (2.5179, 3.0081) ccw
  arc A336 (12.1226, 9.7699) -> (12.2544, 9.8876) centre (11.4288, 10.6792) ccw
  arc A337 (12.1226, 9.7699) -> (12.2544, 9.8876) centre (11.4288, 10.6792) ccw
  line L84 (11.7169, 9.4843) -> (12.1226, 9.7699)
  line L85 (11.7169, 9.4843) -> (12.1226, 9.7699)
  arc A338 (12.8883, 8.8887) -> (12.7257, 8.8196) centre (13.2531, 7.8046) ccw
  arc A339 (13.446, 9.0259) -> (12.8883, 8.8887) centre (13.9153, 5.9163) ccw
  arc A340 (14.5755, 9.0797) -> (13.446, 9.0259) centre (14.2677, 3.6525) ccw
  line L86 (12.2945, 8.5741) -> (12.7257, 8.8196)
  line L87 (12.2945, 8.5741) -> (12.7257, 8.8196)
  arc A341 (12.8883, 8.8887) -> (12.7257, 8.8196) centre (13.2531, 7.8046) ccw
  arc A342 (13.446, 9.0259) -> (12.8883, 8.8887) centre (13.9153, 5.9163) ccw
  arc A343 (14.5755, 9.0797) -> (13.446, 9.0259) centre (14.2677, 3.6525) ccw
  arc A344 (12.2544, 9.8876) -> (12.616, 10.3338) centre (10.0021, 12.0825) ccw
  arc A345 (12.2544, 9.8876) -> (12.616, 10.3338) centre (10.0021, 12.0825) ccw
  arc A346 (12.616, 10.3338) -> (13.1456, 11.333) centre (8.1039, 13.3652) ccw
  arc A347 (13.1456, 11.333) -> (12.6868, 11.8875) centre (2.5179, 3.0081) ccw
  arc A348 (13.1456, 11.333) -> (12.6868, 11.8875) centre (2.5179, 3.0081) ccw
  arc A349 (12.616, 10.3338) -> (13.1456, 11.333) centre (8.1039, 13.3652) ccw
  arc A350 (12.2945, 8.5741) -> (11.7169, 9.4843) centre (2.5179, 3.0081) ccw
  arc A351 (12.2945, 8.5741) -> (11.7169, 9.4843) centre (2.5179, 3.0081) ccw
  arc A352 (10.1393, 11.9461) -> (10.2376, 12.0928) centre (9.2411, 12.6543) ccw
  arc A353 (10.1393, 11.9461) -> (10.2376, 12.0928) centre (9.2411, 12.6543) ccw
  line L88 (9.8174, 11.5685) -> (10.1393, 11.9461)
  line L89 (9.8174, 11.5685) -> (10.1393, 11.9461)
  arc A354 (11.1, 11.283) -> (10.9597, 11.1756) centre (11.7229, 10.3236) ccw
  arc A355 (11.6061, 11.5545) -> (11.1, 11.283) centre (12.834, 8.6593) ccw
  arc A356 (12.6868, 11.8875) -> (11.6061, 11.5545) centre (13.7383, 6.5543) ccw
  line L90 (10.6032, 10.8306) -> (10.9597, 11.1756)
  line L91 (10.6032, 10.8306) -> (10.9597, 11.1756)
  arc A357 (11.1, 11.283) -> (10.9597, 11.1756) centre (11.7229, 10.3236) ccw
  arc A358 (11.6061, 11.5545) -> (11.1, 11.283) centre (12.834, 8.6593) ccw
  arc A359 (12.6868, 11.8875) -> (11.6061, 11.5545) centre (13.7383, 6.5543) ccw
  arc A360 (10.2376, 12.0928) -> (10.4769, 12.6149) centre (7.5103, 13.6586) ccw
  arc A361 (10.2376, 12.0928) -> (10.4769, 12.6149) centre (7.5103, 13.6586) ccw
  arc A362 (10.4769, 12.6149) -> (10.7414, 13.7144) centre (5.3527, 14.429) ccw
  arc A363 (10.7414, 13.7144) -> (10.1591, 14.1374) centre (2.5179, 3.0081) ccw
  arc A364 (10.7414, 13.7144) -> (10.1591, 14.1374) centre (2.5179, 3.0081) ccw
  arc A365 (10.4769, 12.6149) -> (10.7414, 13.7144) centre (5.3527, 14.429) ccw
  arc A366 (10.6032, 10.8306) -> (9.8174, 11.5685) centre (2.5179, 3.0081) ccw
  arc A367 (10.6032, 10.8306) -> (9.8174, 11.5685) centre (2.5179, 3.0081) ccw
  arc A368 (7.6771, 13.5606) -> (7.7358, 13.7272) centre (6.631, 14.0232) ccw
  arc A369 (7.6771, 13.5606) -> (7.7358, 13.7272) centre (6.631, 14.0232) ccw
  line L92 (7.4591, 13.1149) -> (7.6771, 13.5606)
  line L93 (7.4591, 13.1149) -> (7.6771, 13.5606)
  arc A370 (8.7725, 13.1573) -> (8.6633, 13.0184) centre (9.6144, 12.383) ccw
  arc A371 (9.1951, 13.5462) -> (8.7725, 13.1573) centre (11.1045, 11.0473) ccw
  arc A372 (10.1591, 14.1374) -> (9.1951, 13.5462) centre (12.5039, 9.2333) ccw
  line L94 (8.4038, 12.5956) -> (8.6633, 13.0184)
  line L95 (8.4038, 12.5956) -> (8.6633, 13.0184)
  arc A373 (8.7725, 13.1573) -> (8.6633, 13.0184) centre (9.6144, 12.383) ccw
  arc A374 (9.1951, 13.5462) -> (8.7725, 13.1573) centre (11.1045, 11.0473) ccw
  arc A375 (10.1591, 14.1374) -> (9.1951, 13.5462) centre (12.5039, 9.2333) ccw
  arc A376 (7.7358, 13.7272) -> (7.8377, 14.2924) centre (4.7048, 14.5656) ccw
  arc A377 (7.7358, 13.7272) -> (7.8377, 14.2924) centre (4.7048, 14.5656) ccw
  arc A378 (7.8377, 14.2924) -> (7.8205, 15.4231) centre (2.4233, 14.7751) ccw
  arc A379 (7.8205, 15.4231) -> (7.1513, 15.6881) centre (2.5179, 3.0081) ccw
  arc A380 (7.8205, 15.4231) -> (7.1513, 15.6881) centre (2.5179, 3.0081) ccw
  arc A381 (7.8377, 14.2924) -> (7.8205, 15.4231) centre (2.4233, 14.7751) ccw
  arc A382 (8.4038, 12.5956) -> (7.4591, 13.1149) centre (2.5179, 3.0081) ccw
  arc A383 (8.4038, 12.5956) -> (7.4591, 13.1149) centre (2.5179, 3.0081) ccw
  arc A384 (4.8907, 14.5121) -> (4.9061, 14.6881) centre (3.7624, 14.7) ccw
  arc A385 (4.8907, 14.5121) -> (4.9061, 14.6881) centre (3.7624, 14.7) ccw
  line L96 (4.7904, 14.0262) -> (4.8907, 14.5121)
  line L97 (4.7904, 14.0262) -> (4.8907, 14.5121)
  arc A386 (6.052, 14.3939) -> (5.9808, 14.2322) centre (7.06, 13.8533) ccw
  arc A387 (6.3646, 14.8756) -> (6.052, 14.3939) centre (8.8355, 12.9301) ccw
  arc A388 (7.1513, 15.6881) -> (6.3646, 14.8756) centre (10.642, 11.5211) ccw
  line L98 (5.8345, 13.7581) -> (5.9808, 14.2322)
  line L99 (5.8345, 13.7581) -> (5.9808, 14.2322)
  arc A389 (6.052, 14.3939) -> (5.9808, 14.2322) centre (7.06, 13.8533) ccw
  arc A390 (6.3646, 14.8756) -> (6.052, 14.3939) centre (8.8355, 12.9301) ccw
  arc A391 (7.1513, 15.6881) -> (6.3646, 14.8756) centre (10.642, 11.5211) ccw
  arc A392 (4.9061, 14.6881) -> (4.8643, 15.2609) centre (1.7618, 14.7463) ccw
  arc A393 (4.9061, 14.6881) -> (4.8643, 15.2609) centre (1.7618, 14.7463) ccw
  arc A394 (4.8643, 15.2609) -> (4.5664, 16.3518) centre (-0.5, 14.3819) ccw
  arc A395 (4.5664, 16.3518) -> (3.8523, 16.442) centre (2.5179, 3.0081) ccw
  arc A396 (4.5664, 16.3518) -> (3.8523, 16.442) centre (2.5179, 3.0081) ccw
  arc A397 (4.8643, 15.2609) -> (4.5664, 16.3518) centre (-0.5, 14.3819) ccw
  arc A398 (5.8345, 13.7581) -> (4.7904, 14.0262) centre (2.5179, 3.0081) ccw
  arc A399 (5.8345, 13.7581) -> (4.7904, 14.0262) centre (2.5179, 3.0081) ccw
  point P0 (0, 0)
  point P1 (4.8907, 14.5121)
  point P2 (4.9061, 14.6881)
  point P3 (4.8643, 15.2609)
  point P4 (4.5664, 16.3518)
  point P5 (3.8523, 16.442)
  point P6 (3.2924, 15.4594)
  point P7 (3.1095, 14.9151)
  point P8 (3.0807, 14.7407)
  point P9 (1.979, 14.2452)
  point P10 (1.9552, 14.7407)
  point P11 (1.9264, 14.9151)
  point P12 (1.7434, 15.4594)
  point P13 (1.1836, 16.442)
  point P14 (0.4695, 16.3518)
  point P15 (0.1716, 15.2609)
  point P16 (0.1297, 14.6881)
  point P17 (0.1452, 14.5121)
  point P18 (-0.9449, 14.2322)
  point P19 (-1.0161, 14.3939)
  point P20 (-1.3287, 14.8756)
  point P21 (-2.1154, 15.6881)
  point P22 (-2.7846, 15.4231)
  point P23 (-2.8019, 14.2924)
  point P24 (-2.6999, 13.7272)
  point P25 (-2.6412, 13.5606)
  point P26 (-3.6275, 13.0184)
  point P27 (-3.7367, 13.1573)
  point P28 (-4.1592, 13.5462)
  point P29 (-5.1232, 14.1374)
  point P30 (-5.7055, 13.7144)
  point P31 (-5.441, 12.6149)
  point P32 (-5.2017, 12.0928)
  point P33 (-5.1034, 11.9461)
  point P34 (-5.9238, 11.1756)
  point P35 (-6.0642, 11.283)
  point P36 (-6.5702, 11.5545)
  point P37 (-7.6509, 11.8875)
  point P38 (-8.1097, 11.333)
  point P39 (-7.5801, 10.3338)
  point P40 (-7.2185, 9.8876)
  point P41 (-7.0867, 9.7699)
  point P42 (-7.6898, 8.8196)
  point P43 (-7.8524, 8.8887)
  point P44 (-8.4101, 9.0259)
  point P45 (-9.5397, 9.0797)
  point P46 (-9.8461, 8.4284)
  point P47 (-9.0847, 7.5923)
  point P48 (-8.6235, 7.2501)
  point P49 (-8.4666, 7.1689)
  point P50 (-8.8144, 6.0985)
  point P51 (-8.9891, 6.125)
  point P52 (-9.5633, 6.1192)
  point P53 (-10.6708, 5.8903)
  point P54 (-10.8057, 5.1833)
  point P55 (-9.8602, 4.5629)
  point P56 (-9.3284, 4.3461)
  point P57 (-9.1562, 4.3064)
  point P58 (-9.2269, 3.1831)
  point P59 (-9.4027, 3.1654)
  point P60 (-9.9575, 3.0169)
  point P61 (-10.9732, 2.5199)
  point P62 (-10.928, 1.8015)
  point P63 (-9.858, 1.4357)
  point P64 (-9.289, 1.358)
  point P65 (-9.1124, 1.3624)
  point P66 (-8.9015, 0.2568)
  point P67 (-9.0673, 0.1959)
  point P68 (-9.5677, -0.0859)
  point P69 (-10.428, -0.8199)
  point P70 (-10.2056, -1.5044)
  point P71 (-9.0782, -1.5927)
  point P72 (-8.5077, -1.5264)
  point P73 (-8.3377, -1.4783)
  point P74 (-7.8585, -2.4966)
  point P75 (-8.004, -2.5969)
  point P76 (-8.4186, -2.9942)
  point P77 (-9.0693, -3.9192)
  point P78 (-8.6836, -4.5269)
  point P79 (-7.5697, -4.332)
  point P80 (-7.0336, -4.1259)
  point P81 (-6.8809, -4.037)
  point P82 (-6.1635, -4.9042)
  point P83 (-6.2795, -5.0375)
  point P84 (-6.5823, -5.5255)
  point P85 (-6.9825, -6.5832)
  point P86 (-6.4578, -7.0759)
  point P87 (-5.4274, -6.6101)
  point P88 (-4.9594, -6.2772)
  point P89 (-4.8336, -6.1531)
  point P90 (-3.9231, -6.8146)
  point P91 (-4.0023, -6.9726)
  point P92 (-4.1742, -7.5205)
  point P93 (-4.2988, -8.6445)
  point P94 (-3.6681, -8.9912)
  point P95 (-2.7858, -8.2838)
  point P96 (-2.4153, -7.845)
  point P97 (-2.3244, -7.6935)
  point P98 (-1.2779, -8.1078)
  point P99 (-1.3153, -8.2805)
  point P100 (-1.3456, -8.854)
  point P101 (-1.1867, -9.9737)
  point P102 (-0.4896, -10.1526)
  point P103 (0.189, -9.248)
  point P104 (0.4387, -8.7309)
  point P105 (0.4891, -8.5615)
  point P106 (1.6058, -8.7026)
  point P107 (1.6125, -8.8792)
  point P108 (1.7258, -9.4422)
  point P109 (2.1581, -10.4871)
  point P110 (2.8778, -10.4871)
  point P111 (3.3101, -9.4422)
  point P112 (3.4234, -8.8792)
  point P113 (3.4301, -8.7026)
  point P114 (4.5467, -8.5615)
  point P115 (4.5971, -8.7309)
  point P116 (4.8469, -9.248)
  point P117 (5.5255, -10.1526)
  point P118 (6.2226, -9.9737)
  point P119 (6.3815, -8.854)
  point P120 (6.3512, -8.2805)
  point P121 (6.3138, -8.1078)
  point P122 (7.3603, -7.6935)
  point P123 (7.4512, -7.845)
  point P124 (7.8217, -8.2838)
  point P125 (8.704, -8.9912)
  point P126 (9.3347, -8.6445)
  point P127 (9.2101, -7.5205)
  point P128 (9.0381, -6.9726)
  point P129 (8.959, -6.8146)
  point P130 (9.8695, -6.1531)
  point P131 (9.9953, -6.2772)
  point P132 (10.4633, -6.6101)
  point P133 (11.4937, -7.0759)
  point P134 (12.0184, -6.5832)
  point P135 (11.6182, -5.5255)
  point P136 (11.3154, -5.0375)
  point P137 (11.1994, -4.9042)
  point P138 (11.9168, -4.037)
  point P139 (12.0695, -4.1259)
  point P140 (12.6056, -4.332)
  point P141 (13.7195, -4.5269)
  point P142 (14.1051, -3.9192)
  point P143 (13.4545, -2.9942)
  point P144 (13.0399, -2.5969)
  point P145 (12.8944, -2.4966)
  point P146 (13.3736, -1.4783)
  point P147 (13.5436, -1.5264)
  point P148 (14.114, -1.5927)
  point P149 (15.2414, -1.5044)
  point P150 (15.4638, -0.8199)
  point P151 (14.6036, -0.0859)
  point P152 (14.1032, 0.1959)
  point P153 (13.9373, 0.2568)
  point P154 (14.1482, 1.3624)
  point P155 (14.3249, 1.358)
  point P156 (14.8939, 1.4357)
  point P157 (15.9639, 1.8015)
  point P158 (16.0091, 2.5199)
  point P159 (14.9934, 3.0169)
  point P160 (14.4386, 3.1654)
  point P161 (14.2628, 3.1831)
  point P162 (14.1921, 4.3064)
  point P163 (14.3643, 4.3461)
  point P164 (14.8961, 4.5629)
  point P165 (15.8415, 5.1833)
  point P166 (15.7067, 5.8903)
  point P167 (14.5992, 6.1192)
  point P168 (14.025, 6.125)
  point P169 (13.8503, 6.0985)
  point P170 (13.5025, 7.1689)
  point P171 (13.6594, 7.2501)
  point P172 (14.1206, 7.5923)
  point P173 (14.882, 8.4284)
  point P174 (14.5755, 9.0797)
  point P175 (13.446, 9.0259)
  point P176 (12.8883, 8.8887)
  point P177 (12.7257, 8.8196)
  point P178 (12.1226, 9.7699)
  point P179 (12.2544, 9.8876)
  point P180 (12.616, 10.3338)
  point P181 (13.1456, 11.333)
  point P182 (12.6868, 11.8875)
  point P183 (11.6061, 11.5545)
  point P184 (11.1, 11.283)
  point P185 (10.9597, 11.1756)
  point P186 (10.1393, 11.9461)
  point P187 (10.2376, 12.0928)
  point P188 (10.4769, 12.6149)
  point P189 (10.7414, 13.7144)
  point P190 (10.1591, 14.1374)
  point P191 (9.1951, 13.5462)
  point P192 (8.7725, 13.1573)
  point P193 (8.6633, 13.0184)
  point P194 (7.6771, 13.5606)
  point P195 (7.7358, 13.7272)
  point P196 (7.8377, 14.2924)
  point P197 (7.8205, 15.4231)
  point P198 (7.1513, 15.6881)
  point P199 (6.3646, 14.8756)
  dimension "d2" = 360
  constraints: 800 point on circle, 400 centre point, 200 end point, 2 coincident, 1899 other
extrude "押し出し1" add sketch "スケッチ1" along normal blind 8
